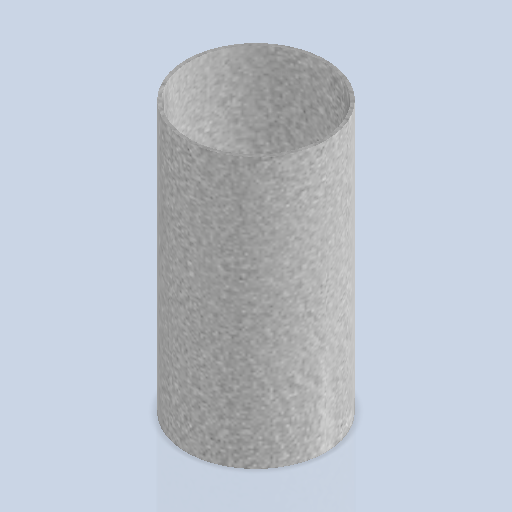
# Autodesk Inventor part: cylinder
Saved by Autodesk Inventor 2024.2 (Build 282272000, 272)
## iProperties
Created: 2024-05-05
Part Number: cylinder
Material: Glasfaserbeton
Document SubType Name: Modeling
Designer: Fabri
Density: 1.7 g/cm^3
Appearance: Flach - Poliert Grau
Author: Fabri
Autodesk Inventor part; units mm, degrees
ref_plane "YZ Plane" through (0, 0, 0) normal (1, 0, 0) x (0, 1, 0)
ref_plane "XZ Plane" through (0, 0, 0) normal (0, 1, 0) x (-1, 0, 0)
ref_plane "XY Plane" through (0, 0, 0) normal (0, 0, 1) x (1, 0, 0)
sketch "Skizze1" plane through (0, 0, 0) normal (0, 1, 0) x (-1, 0, 0)
  line L0 (0, 0) -> (33, 0)
  line L1 (33, 0) -> (33, -3)
  line L2 (33, -127.5) -> (0, -127.5)
  line L3 (0, -127.5) -> (0, 0)
  line L4 (33, -3) -> (33, -127.5)
  dimension "d0" = 127.5
  dimension "d4" = 66
  constraints: 10 end point, 2 perpendicular, 1 horizontal, 1 point on line
  measures "d0" distance between parallel lines of L2 L0
  measures "d4" diameter of L4 L3
revolve "Umdrehung1" add sketch "Skizze1" angle 360 about axis through (0, 0, -127.5) along (0, 0, 1)
sketch "Skizze3" plane through (0, 0, -127.5) normal (0, 0, -1) x (-1, 0, 0)
  circle A0 centre (0, 0) radius 31.5
  point P0 (0, 0)
  dimension "d7" = 63
  constraints: 1 centre point, 1 coincident
  measures "d7" diameter of A0
extrude "Extrusion1" cut sketch "Skizze3" against normal up to surface (127.5 mm away)
